Autodesk Fusion 360 part; units mm, degrees
(part 2 of 3)
sketch "스케치11" plane through (120.25, 0, 0) normal (1, 0, 0) x (0, 1, 0)
  line L0 (-4, 0) -> (79.3, 0)
  line L1 (79.3, 0) -> (79.3, 132.5)
  line L2 (79.3, 132.5) -> (-4, 132.5)
  line L3 (-4, 132.5) -> (-4, 0)
  line L4 (1, 128.5) -> (1, 4)
  line L5 (1, 4) -> (74.3, 4)
  line L6 (74.3, 4) -> (74.3, 128.5)
  line L7 (74.3, 128.5) -> (1, 128.5)
  line L8 (40.15, 61.9199) -> (42.65, 66.25)
  line L9 (42.65, 66.25) -> (40.15, 70.5801)
  line L10 (40.15, 70.5801) -> (35.15, 70.5801)
  line L11 (35.15, 70.5801) -> (32.65, 66.25)
  line L12 (32.65, 66.25) -> (35.15, 61.9199)
  line L13 (35.15, 61.9199) -> (40.15, 61.9199)
  line L14 (51.8821, 60.9199) -> (49.3821, 65.25)
  line L15 (49.3821, 65.25) -> (44.3821, 65.25)
  line L16 (44.3821, 65.25) -> (41.8821, 60.9199)
  line L17 (41.8821, 60.9199) -> (44.3821, 56.5897)
  line L18 (44.3821, 56.5897) -> (49.3821, 56.5897)
  line L19 (49.3821, 56.5897) -> (51.8821, 60.9199)
  line L20 (42.65, 66.25) -> (44.3821, 65.25) construction
  line L21 (74.3, 66.25) -> (1, 66.25) construction
  line L22 (37.65, 128.5) -> (37.65, 4) construction
  line L23 (-4, 132.5) -> (-4, 0)
  line L24 (79.3, 132.5) -> (79.3, 0)
  line L25 (79.3, 132.5) -> (-4, 132.5)
  line L26 (5.722, 2.29) -> (3.222, 6.6201)
  line L27 (7.4541, 1.29) -> (4.9541, -3.0401)
  line L28 (3.222, -2.0401) -> (5.722, 2.29)
  line L29 (3.222, 6.6201) -> (-1.778, 6.6201)
  line L30 (14.9541, -3.0401) -> (12.4541, 1.29)
  line L31 (12.4541, 1.29) -> (7.4541, 1.29)
  line L32 (7.4541, -7.3703) -> (12.4541, -7.3703)
  line L33 (12.4541, -7.3703) -> (14.9541, -3.0401)
  line L34 (-1.778, -2.0401) -> (3.222, -2.0401)
  line L35 (4.9541, -3.0401) -> (7.4541, -7.3703)
  line L36 (-1.778, 6.6201) -> (-4.278, 2.29)
  line L37 (-4.278, 2.29) -> (-1.778, -2.0401)
  line L38 (5.722, 2.29) -> (7.4541, 1.29) construction
  line L39 (24.186, 2.29) -> (21.686, 6.6201)
  line L40 (25.9181, 1.29) -> (23.4181, -3.0401)
  line L41 (21.686, -2.0401) -> (24.186, 2.29)
  line L42 (21.686, 6.6201) -> (16.686, 6.6201)
  line L43 (33.4181, -3.0401) -> (30.9181, 1.29)
  line L44 (30.9181, 1.29) -> (25.9181, 1.29)
  line L45 (25.9181, -7.3703) -> (30.9181, -7.3703)
  line L46 (30.9181, -7.3703) -> (33.4181, -3.0401)
  line L47 (16.686, -2.0401) -> (21.686, -2.0401)
  line L48 (23.4181, -3.0401) -> (25.9181, -7.3703)
  line L49 (16.686, 6.6201) -> (14.186, 2.29)
  line L50 (14.186, 2.29) -> (16.686, -2.0401)
  line L51 (24.186, 2.29) -> (25.9181, 1.29) construction
  line L52 (42.65, 2.29) -> (40.15, 6.6201)
  line L53 (44.3821, 1.29) -> (41.8821, -3.0401)
  line L54 (40.15, -2.0401) -> (42.65, 2.29)
  line L55 (40.15, 6.6201) -> (35.15, 6.6201)
  line L56 (51.8821, -3.0401) -> (49.3821, 1.29)
  line L57 (49.3821, 1.29) -> (44.3821, 1.29)
  line L58 (44.3821, -7.3703) -> (49.3821, -7.3703)
  line L59 (49.3821, -7.3703) -> (51.8821, -3.0401)
  line L60 (35.15, -2.0401) -> (40.15, -2.0401)
  line L61 (41.8821, -3.0401) -> (44.3821, -7.3703)
  line L62 (35.15, 6.6201) -> (32.65, 2.29)
  line L63 (32.65, 2.29) -> (35.15, -2.0401)
  line L64 (42.65, 2.29) -> (44.3821, 1.29) construction
  line L65 (61.114, 2.29) -> (58.614, 6.6201)
  line L66 (62.8461, 1.29) -> (60.3461, -3.0401)
  line L67 (58.614, -2.0401) -> (61.114, 2.29)
  line L68 (58.614, 6.6201) -> (53.614, 6.6201)
  line L69 (70.3461, -3.0401) -> (67.8461, 1.29)
  line L70 (67.8461, 1.29) -> (62.8461, 1.29)
  line L71 (62.8461, -7.3703) -> (67.8461, -7.3703)
  line L72 (67.8461, -7.3703) -> (70.3461, -3.0401)
  line L73 (53.614, -2.0401) -> (58.614, -2.0401)
  line L74 (60.3461, -3.0401) -> (62.8461, -7.3703)
  line L75 (53.614, 6.6201) -> (51.114, 2.29)
  line L76 (51.114, 2.29) -> (53.614, -2.0401)
  line L77 (61.114, 2.29) -> (62.8461, 1.29) construction
  line L78 (79.578, 2.29) -> (77.078, 6.6201)
  line L79 (81.3101, 1.29) -> (78.8101, -3.0401)
  line L80 (77.078, -2.0401) -> (79.578, 2.29)
  line L81 (77.078, 6.6201) -> (72.078, 6.6201)
  line L82 (88.8101, -3.0401) -> (86.3101, 1.29)
  line L83 (86.3101, 1.29) -> (81.3101, 1.29)
  line L84 (81.3101, -7.3703) -> (86.3101, -7.3703)
  line L85 (86.3101, -7.3703) -> (88.8101, -3.0401)
  line L86 (72.078, -2.0401) -> (77.078, -2.0401)
  line L87 (78.8101, -3.0401) -> (81.3101, -7.3703)
  line L88 (72.078, 6.6201) -> (69.578, 2.29)
  line L89 (69.578, 2.29) -> (72.078, -2.0401)
  line L90 (79.578, 2.29) -> (81.3101, 1.29) construction
  line L91 (5.722, 12.95) -> (3.222, 17.2801)
  line L92 (7.4541, 11.95) -> (4.9541, 7.6199)
  line L93 (3.222, 8.6199) -> (5.722, 12.95)
  line L94 (3.222, 17.2801) -> (-1.778, 17.2801)
  line L95 (14.9541, 7.6199) -> (12.4541, 11.95)
  line L96 (12.4541, 11.95) -> (7.4541, 11.95)
  line L97 (7.4541, 3.2897) -> (12.4541, 3.2897)
  line L98 (12.4541, 3.2897) -> (14.9541, 7.6199)
  line L99 (-1.778, 8.6199) -> (3.222, 8.6199)
  line L100 (4.9541, 7.6199) -> (7.4541, 3.2897)
  line L101 (-1.778, 17.2801) -> (-4.278, 12.95)
  line L102 (-4.278, 12.95) -> (-1.778, 8.6199)
  line L103 (5.722, 12.95) -> (7.4541, 11.95) construction
  line L104 (24.186, 12.95) -> (21.686, 17.2801)
  line L105 (25.9181, 11.95) -> (23.4181, 7.6199)
  line L106 (21.686, 8.6199) -> (24.186, 12.95)
  line L107 (21.686, 17.2801) -> (16.686, 17.2801)
  line L108 (33.4181, 7.6199) -> (30.9181, 11.95)
  line L109 (30.9181, 11.95) -> (25.9181, 11.95)
  line L110 (25.9181, 3.2897) -> (30.9181, 3.2897)
  line L111 (30.9181, 3.2897) -> (33.4181, 7.6199)
  line L112 (16.686, 8.6199) -> (21.686, 8.6199)
  line L113 (23.4181, 7.6199) -> (25.9181, 3.2897)
  line L114 (16.686, 17.2801) -> (14.186, 12.95)
  line L115 (14.186, 12.95) -> (16.686, 8.6199)
  line L116 (24.186, 12.95) -> (25.9181, 11.95) construction
  line L117 (42.65, 12.95) -> (40.15, 17.2801)
  line L118 (44.3821, 11.95) -> (41.8821, 7.6199)
  line L119 (40.15, 8.6199) -> (42.65, 12.95)
  line L120 (40.15, 17.2801) -> (35.15, 17.2801)
  line L121 (51.8821, 7.6199) -> (49.3821, 11.95)
  line L122 (49.3821, 11.95) -> (44.3821, 11.95)
  line L123 (44.3821, 3.2897) -> (49.3821, 3.2897)
  line L124 (49.3821, 3.2897) -> (51.8821, 7.6199)
  line L125 (35.15, 8.6199) -> (40.15, 8.6199)
  line L126 (41.8821, 7.6199) -> (44.3821, 3.2897)
  line L127 (35.15, 17.2801) -> (32.65, 12.95)
  line L128 (32.65, 12.95) -> (35.15, 8.6199)
  line L129 (42.65, 12.95) -> (44.3821, 11.95) construction
  line L130 (61.114, 12.95) -> (58.614, 17.2801)
  line L131 (62.8461, 11.95) -> (60.3461, 7.6199)
  line L132 (58.614, 8.6199) -> (61.114, 12.95)
  line L133 (58.614, 17.2801) -> (53.614, 17.2801)
  line L134 (70.3461, 7.6199) -> (67.8461, 11.95)
  line L135 (67.8461, 11.95) -> (62.8461, 11.95)
  line L136 (62.8461, 3.2897) -> (67.8461, 3.2897)
  line L137 (67.8461, 3.2897) -> (70.3461, 7.6199)
  line L138 (53.614, 8.6199) -> (58.614, 8.6199)
  line L139 (60.3461, 7.6199) -> (62.8461, 3.2897)
  line L140 (53.614, 17.2801) -> (51.114, 12.95)
  line L141 (51.114, 12.95) -> (53.614, 8.6199)
  line L142 (61.114, 12.95) -> (62.8461, 11.95) construction
  line L143 (79.578, 12.95) -> (77.078, 17.2801)
  line L144 (81.3101, 11.95) -> (78.8101, 7.6199)
  line L145 (77.078, 8.6199) -> (79.578, 12.95)
  line L146 (77.078, 17.2801) -> (72.078, 17.2801)
  line L147 (88.8101, 7.6199) -> (86.3101, 11.95)
  line L148 (86.3101, 11.95) -> (81.3101, 11.95)
  line L149 (81.3101, 3.2897) -> (86.3101, 3.2897)
  line L150 (86.3101, 3.2897) -> (88.8101, 7.6199)
  line L151 (72.078, 8.6199) -> (77.078, 8.6199)
  line L152 (78.8101, 7.6199) -> (81.3101, 3.2897)
  line L153 (72.078, 17.2801) -> (69.578, 12.95)
  line L154 (69.578, 12.95) -> (72.078, 8.6199)
  line L155 (79.578, 12.95) -> (81.3101, 11.95) construction
  line L156 (5.722, 23.61) -> (3.222, 27.9401)
  line L157 (7.4541, 22.61) -> (4.9541, 18.2799)
  line L158 (3.222, 19.2799) -> (5.722, 23.61)
  line L159 (3.222, 27.9401) -> (-1.778, 27.9401)
  line L160 (14.9541, 18.2799) -> (12.4541, 22.61)
  line L161 (12.4541, 22.61) -> (7.4541, 22.61)
  line L162 (7.4541, 13.9497) -> (12.4541, 13.9497)
  line L163 (12.4541, 13.9497) -> (14.9541, 18.2799)
  line L164 (-1.778, 19.2799) -> (3.222, 19.2799)
  line L165 (4.9541, 18.2799) -> (7.4541, 13.9497)
  line L166 (-1.778, 27.9401) -> (-4.278, 23.61)
  line L167 (-4.278, 23.61) -> (-1.778, 19.2799)
  line L168 (5.722, 23.61) -> (7.4541, 22.61) construction
  line L169 (24.186, 23.61) -> (21.686, 27.9401)
  line L170 (25.9181, 22.61) -> (23.4181, 18.2799)
  line L171 (21.686, 19.2799) -> (24.186, 23.61)
  line L172 (21.686, 27.9401) -> (16.686, 27.9401)
  line L173 (33.4181, 18.2799) -> (30.9181, 22.61)
  line L174 (30.9181, 22.61) -> (25.9181, 22.61)
  line L175 (25.9181, 13.9497) -> (30.9181, 13.9497)
  line L176 (30.9181, 13.9497) -> (33.4181, 18.2799)
  line L177 (16.686, 19.2799) -> (21.686, 19.2799)
  line L178 (23.4181, 18.2799) -> (25.9181, 13.9497)
  line L179 (16.686, 27.9401) -> (14.186, 23.61)
  line L180 (14.186, 23.61) -> (16.686, 19.2799)
  line L181 (24.186, 23.61) -> (25.9181, 22.61) construction
  line L182 (42.65, 23.61) -> (40.15, 27.9401)
  line L183 (44.3821, 22.61) -> (41.8821, 18.2799)
  line L184 (40.15, 19.2799) -> (42.65, 23.61)
  line L185 (40.15, 27.9401) -> (35.15, 27.9401)
  line L186 (51.8821, 18.2799) -> (49.3821, 22.61)
  line L187 (49.3821, 22.61) -> (44.3821, 22.61)
  line L188 (44.3821, 13.9497) -> (49.3821, 13.9497)
  line L189 (49.3821, 13.9497) -> (51.8821, 18.2799)
  line L190 (35.15, 19.2799) -> (40.15, 19.2799)
  line L191 (41.8821, 18.2799) -> (44.3821, 13.9497)
  line L192 (35.15, 27.9401) -> (32.65, 23.61)
  line L193 (32.65, 23.61) -> (35.15, 19.2799)
  line L194 (42.65, 23.61) -> (44.3821, 22.61) construction
  line L195 (61.114, 23.61) -> (58.614, 27.9401)
  line L196 (62.8461, 22.61) -> (60.3461, 18.2799)
  line L197 (58.614, 19.2799) -> (61.114, 23.61)
  line L198 (58.614, 27.9401) -> (53.614, 27.9401)
  line L199 (70.3461, 18.2799) -> (67.8461, 22.61)
  line L200 (67.8461, 22.61) -> (62.8461, 22.61)
  line L201 (62.8461, 13.9497) -> (67.8461, 13.9497)
  line L202 (67.8461, 13.9497) -> (70.3461, 18.2799)
  line L203 (53.614, 19.2799) -> (58.614, 19.2799)
  line L204 (60.3461, 18.2799) -> (62.8461, 13.9497)
  line L205 (53.614, 27.9401) -> (51.114, 23.61)
  line L206 (51.114, 23.61) -> (53.614, 19.2799)
  line L207 (61.114, 23.61) -> (62.8461, 22.61) construction
  line L208 (79.578, 23.61) -> (77.078, 27.9401)
  line L209 (81.3101, 22.61) -> (78.8101, 18.2799)
  line L210 (77.078, 19.2799) -> (79.578, 23.61)
  line L211 (77.078, 27.9401) -> (72.078, 27.9401)
  line L212 (88.8101, 18.2799) -> (86.3101, 22.61)
  line L213 (86.3101, 22.61) -> (81.3101, 22.61)
  line L214 (81.3101, 13.9497) -> (86.3101, 13.9497)
  line L215 (86.3101, 13.9497) -> (88.8101, 18.2799)
  line L216 (72.078, 19.2799) -> (77.078, 19.2799)
  line L217 (78.8101, 18.2799) -> (81.3101, 13.9497)
  line L218 (72.078, 27.9401) -> (69.578, 23.61)
  line L219 (69.578, 23.61) -> (72.078, 19.2799)
  line L220 (79.578, 23.61) -> (81.3101, 22.61) construction
  line L221 (5.722, 34.27) -> (3.222, 38.6001)
  line L222 (7.4541, 33.27) -> (4.9541, 28.9399)
  line L223 (3.222, 29.9399) -> (5.722, 34.27)
  line L224 (3.222, 38.6001) -> (-1.778, 38.6001)
  line L225 (14.9541, 28.9399) -> (12.4541, 33.27)
  line L226 (12.4541, 33.27) -> (7.4541, 33.27)
  line L227 (7.4541, 24.6097) -> (12.4541, 24.6097)
  line L228 (12.4541, 24.6097) -> (14.9541, 28.9399)
  line L229 (-1.778, 29.9399) -> (3.222, 29.9399)
  line L230 (4.9541, 28.9399) -> (7.4541, 24.6097)
  line L231 (-1.778, 38.6001) -> (-4.278, 34.27)
  line L232 (-4.278, 34.27) -> (-1.778, 29.9399)
  line L233 (5.722, 34.27) -> (7.4541, 33.27) construction
  line L234 (24.186, 34.27) -> (21.686, 38.6001)
  line L235 (25.9181, 33.27) -> (23.4181, 28.9399)
  line L236 (21.686, 29.9399) -> (24.186, 34.27)
  line L237 (21.686, 38.6001) -> (16.686, 38.6001)
  line L238 (33.4181, 28.9399) -> (30.9181, 33.27)
  line L239 (30.9181, 33.27) -> (25.9181, 33.27)
  line L240 (25.9181, 24.6097) -> (30.9181, 24.6097)
  line L241 (30.9181, 24.6097) -> (33.4181, 28.9399)
  line L242 (16.686, 29.9399) -> (21.686, 29.9399)
  line L243 (23.4181, 28.9399) -> (25.9181, 24.6097)
  line L244 (16.686, 38.6001) -> (14.186, 34.27)
  line L245 (14.186, 34.27) -> (16.686, 29.9399)
  line L246 (24.186, 34.27) -> (25.9181, 33.27) construction
  line L247 (42.65, 34.27) -> (40.15, 38.6001)
  line L248 (44.3821, 33.27) -> (41.8821, 28.9399)
  line L249 (40.15, 29.9399) -> (42.65, 34.27)
  line L250 (40.15, 38.6001) -> (35.15, 38.6001)
  line L251 (51.8821, 28.9399) -> (49.3821, 33.27)
  line L252 (49.3821, 33.27) -> (44.3821, 33.27)
  line L253 (44.3821, 24.6097) -> (49.3821, 24.6097)
  line L254 (49.3821, 24.6097) -> (51.8821, 28.9399)
  line L255 (35.15, 29.9399) -> (40.15, 29.9399)
  line L256 (41.8821, 28.9399) -> (44.3821, 24.6097)
  line L257 (35.15, 38.6001) -> (32.65, 34.27)
  line L258 (32.65, 34.27) -> (35.15, 29.9399)
  line L259 (42.65, 34.27) -> (44.3821, 33.27) construction
  line L260 (61.114, 34.27) -> (58.614, 38.6001)
  line L261 (62.8461, 33.27) -> (60.3461, 28.9399)
  line L262 (58.614, 29.9399) -> (61.114, 34.27)
  line L263 (58.614, 38.6001) -> (53.614, 38.6001)
  line L264 (70.3461, 28.9399) -> (67.8461, 33.27)
  line L265 (67.8461, 33.27) -> (62.8461, 33.27)
  line L266 (62.8461, 24.6097) -> (67.8461, 24.6097)
  line L267 (67.8461, 24.6097) -> (70.3461, 28.9399)
  line L268 (53.614, 29.9399) -> (58.614, 29.9399)
  line L269 (60.3461, 28.9399) -> (62.8461, 24.6097)
  line L270 (53.614, 38.6001) -> (51.114, 34.27)
  line L271 (51.114, 34.27) -> (53.614, 29.9399)
  line L272 (61.114, 34.27) -> (62.8461, 33.27) construction
  line L273 (79.578, 34.27) -> (77.078, 38.6001)
  line L274 (81.3101, 33.27) -> (78.8101, 28.9399)
  line L275 (77.078, 29.9399) -> (79.578, 34.27)
  line L276 (77.078, 38.6001) -> (72.078, 38.6001)
  line L277 (88.8101, 28.9399) -> (86.3101, 33.27)
  line L278 (86.3101, 33.27) -> (81.3101, 33.27)
  line L279 (81.3101, 24.6097) -> (86.3101, 24.6097)
  line L280 (86.3101, 24.6097) -> (88.8101, 28.9399)
  line L281 (72.078, 29.9399) -> (77.078, 29.9399)
  line L282 (78.8101, 28.9399) -> (81.3101, 24.6097)
  line L283 (72.078, 38.6001) -> (69.578, 34.27)
  line L284 (69.578, 34.27) -> (72.078, 29.9399)
  line L285 (79.578, 34.27) -> (81.3101, 33.27) construction
  line L286 (5.722, 44.93) -> (3.222, 49.2601)
  line L287 (7.4541, 43.93) -> (4.9541, 39.5999)
  line L288 (3.222, 40.5999) -> (5.722, 44.93)
  line L289 (3.222, 49.2601) -> (-1.778, 49.2601)
  line L290 (14.9541, 39.5999) -> (12.4541, 43.93)
  line L291 (12.4541, 43.93) -> (7.4541, 43.93)
  line L292 (7.4541, 35.2697) -> (12.4541, 35.2697)
  line L293 (12.4541, 35.2697) -> (14.9541, 39.5999)
  line L294 (-1.778, 40.5999) -> (3.222, 40.5999)
  line L295 (4.9541, 39.5999) -> (7.4541, 35.2697)
  line L296 (-1.778, 49.2601) -> (-4.278, 44.93)
  line L297 (-4.278, 44.93) -> (-1.778, 40.5999)
  line L298 (5.722, 44.93) -> (7.4541, 43.93) construction
  line L299 (24.186, 44.93) -> (21.686, 49.2601)
  line L300 (25.9181, 43.93) -> (23.4181, 39.5999)
  line L301 (21.686, 40.5999) -> (24.186, 44.93)
  line L302 (21.686, 49.2601) -> (16.686, 49.2601)
  line L303 (33.4181, 39.5999) -> (30.9181, 43.93)
  line L304 (30.9181, 43.93) -> (25.9181, 43.93)
  line L305 (25.9181, 35.2697) -> (30.9181, 35.2697)
  line L306 (30.9181, 35.2697) -> (33.4181, 39.5999)
  line L307 (16.686, 40.5999) -> (21.686, 40.5999)
  line L308 (23.4181, 39.5999) -> (25.9181, 35.2697)
  line L309 (16.686, 49.2601) -> (14.186, 44.93)
  line L310 (14.186, 44.93) -> (16.686, 40.5999)
  line L311 (24.186, 44.93) -> (25.9181, 43.93) construction
  line L312 (42.65, 44.93) -> (40.15, 49.2601)
  line L313 (44.3821, 43.93) -> (41.8821, 39.5999)
  line L314 (40.15, 40.5999) -> (42.65, 44.93)
  line L315 (40.15, 49.2601) -> (35.15, 49.2601)
  line L316 (51.8821, 39.5999) -> (49.3821, 43.93)
  line L317 (49.3821, 43.93) -> (44.3821, 43.93)
  line L318 (44.3821, 35.2697) -> (49.3821, 35.2697)
  line L319 (49.3821, 35.2697) -> (51.8821, 39.5999)
  line L320 (35.15, 40.5999) -> (40.15, 40.5999)
  line L321 (41.8821, 39.5999) -> (44.3821, 35.2697)
  line L322 (35.15, 49.2601) -> (32.65, 44.93)
  line L323 (32.65, 44.93) -> (35.15, 40.5999)
  line L324 (42.65, 44.93) -> (44.3821, 43.93) construction
  line L325 (61.114, 44.93) -> (58.614, 49.2601)
  line L326 (62.8461, 43.93) -> (60.3461, 39.5999)
  line L327 (58.614, 40.5999) -> (61.114, 44.93)
  line L328 (58.614, 49.2601) -> (53.614, 49.2601)
  line L329 (70.3461, 39.5999) -> (67.8461, 43.93)
  line L330 (67.8461, 43.93) -> (62.8461, 43.93)
  line L331 (62.8461, 35.2697) -> (67.8461, 35.2697)
  line L332 (67.8461, 35.2697) -> (70.3461, 39.5999)
  line L333 (53.614, 40.5999) -> (58.614, 40.5999)
  line L334 (60.3461, 39.5999) -> (62.8461, 35.2697)
  line L335 (53.614, 49.2601) -> (51.114, 44.93)
  line L336 (51.114, 44.93) -> (53.614, 40.5999)
  line L337 (61.114, 44.93) -> (62.8461, 43.93) construction
  line L338 (79.578, 44.93) -> (77.078, 49.2601)
  line L339 (81.3101, 43.93) -> (78.8101, 39.5999)
  line L340 (77.078, 40.5999) -> (79.578, 44.93)
  line L341 (77.078, 49.2601) -> (72.078, 49.2601)
  line L342 (88.8101, 39.5999) -> (86.3101, 43.93)
  line L343 (86.3101, 43.93) -> (81.3101, 43.93)
  line L344 (81.3101, 35.2697) -> (86.3101, 35.2697)
  line L345 (86.3101, 35.2697) -> (88.8101, 39.5999)
  line L346 (72.078, 40.5999) -> (77.078, 40.5999)
  line L347 (78.8101, 39.5999) -> (81.3101, 35.2697)
  line L348 (72.078, 49.2601) -> (69.578, 44.93)
  line L349 (69.578, 44.93) -> (72.078, 40.5999)
  line L350 (79.578, 44.93) -> (81.3101, 43.93) construction
  line L351 (5.722, 55.59) -> (3.222, 59.9201)
  line L352 (7.4541, 54.59) -> (4.9541, 50.2599)
  line L353 (3.222, 51.2599) -> (5.722, 55.59)
  line L354 (3.222, 59.9201) -> (-1.778, 59.9201)
  line L355 (14.9541, 50.2599) -> (12.4541, 54.59)
  line L356 (12.4541, 54.59) -> (7.4541, 54.59)
  line L357 (7.4541, 45.9297) -> (12.4541, 45.9297)
  line L358 (12.4541, 45.9297) -> (14.9541, 50.2599)
  line L359 (-1.778, 51.2599) -> (3.222, 51.2599)
  line L360 (4.9541, 50.2599) -> (7.4541, 45.9297)
  line L361 (-1.778, 59.9201) -> (-4.278, 55.59)
  line L362 (-4.278, 55.59) -> (-1.778, 51.2599)
  line L363 (5.722, 55.59) -> (7.4541, 54.59) construction
  line L364 (24.186, 55.59) -> (21.686, 59.9201)
  line L365 (25.9181, 54.59) -> (23.4181, 50.2599)
  line L366 (21.686, 51.2599) -> (24.186, 55.59)
  line L367 (21.686, 59.9201) -> (16.686, 59.9201)
  line L368 (33.4181, 50.2599) -> (30.9181, 54.59)
  line L369 (30.9181, 54.59) -> (25.9181, 54.59)
  line L370 (25.9181, 45.9297) -> (30.9181, 45.9297)
  line L371 (30.9181, 45.9297) -> (33.4181, 50.2599)
  line L372 (16.686, 51.2599) -> (21.686, 51.2599)
  line L373 (23.4181, 50.2599) -> (25.9181, 45.9297)
  line L374 (16.686, 59.9201) -> (14.186, 55.59)
  line L375 (14.186, 55.59) -> (16.686, 51.2599)
  line L376 (24.186, 55.59) -> (25.9181, 54.59) construction
  line L377 (42.65, 55.59) -> (40.15, 59.9201)
  line L378 (44.3821, 54.59) -> (41.8821, 50.2599)
  line L379 (40.15, 51.2599) -> (42.65, 55.59)
  line L380 (40.15, 59.9201) -> (35.15, 59.9201)
  line L381 (51.8821, 50.2599) -> (49.3821, 54.59)
  line L382 (49.3821, 54.59) -> (44.3821, 54.59)
  line L383 (44.3821, 45.9297) -> (49.3821, 45.9297)
  line L384 (49.3821, 45.9297) -> (51.8821, 50.2599)
  line L385 (35.15, 51.2599) -> (40.15, 51.2599)
  line L386 (41.8821, 50.2599) -> (44.3821, 45.9297)
  line L387 (35.15, 59.9201) -> (32.65, 55.59)
  line L388 (32.65, 55.59) -> (35.15, 51.2599)
  line L389 (42.65, 55.59) -> (44.3821, 54.59) construction
  line L390 (61.114, 55.59) -> (58.614, 59.9201)
  line L391 (62.8461, 54.59) -> (60.3461, 50.2599)
  line L392 (58.614, 51.2599) -> (61.114, 55.59)
  line L393 (58.614, 59.9201) -> (53.614, 59.9201)
  line L394 (70.3461, 50.2599) -> (67.8461, 54.59)
  line L395 (67.8461, 54.59) -> (62.8461, 54.59)
  line L396 (62.8461, 45.9297) -> (67.8461, 45.9297)
  line L397 (67.8461, 45.9297) -> (70.3461, 50.2599)
  line L398 (53.614, 51.2599) -> (58.614, 51.2599)
  line L399 (60.3461, 50.2599) -> (62.8461, 45.9297)
  line L400 (53.614, 59.9201) -> (51.114, 55.59)
  line L401 (51.114, 55.59) -> (53.614, 51.2599)
  line L402 (61.114, 55.59) -> (62.8461, 54.59) construction
  line L403 (79.578, 55.59) -> (77.078, 59.9201)
  line L404 (81.3101, 54.59) -> (78.8101, 50.2599)
  line L405 (77.078, 51.2599) -> (79.578, 55.59)
  line L406 (77.078, 59.9201) -> (72.078, 59.9201)
  line L407 (88.8101, 50.2599) -> (86.3101, 54.59)
  line L408 (86.3101, 54.59) -> (81.3101, 54.59)
  line L409 (81.3101, 45.9297) -> (86.3101, 45.9297)
  line L410 (86.3101, 45.9297) -> (88.8101, 50.2599)
  line L411 (72.078, 51.2599) -> (77.078, 51.2599)
  line L412 (78.8101, 50.2599) -> (81.3101, 45.9297)
  line L413 (72.078, 59.9201) -> (69.578, 55.59)
  line L414 (69.578, 55.59) -> (72.078, 51.2599)
  line L415 (79.578, 55.59) -> (81.3101, 54.59) construction
  line L416 (5.722, 66.25) -> (3.222, 70.5801)
  line L417 (7.4541, 65.25) -> (4.9541, 60.9199)
  line L418 (3.222, 61.9199) -> (5.722, 66.25)
  line L419 (3.222, 70.5801) -> (-1.778, 70.5801)
  line L420 (14.9541, 60.9199) -> (12.4541, 65.25)
  line L421 (12.4541, 65.25) -> (7.4541, 65.25)
  line L422 (7.4541, 56.5897) -> (12.4541, 56.5897)
  line L423 (12.4541, 56.5897) -> (14.9541, 60.9199)
  line L424 (-1.778, 61.9199) -> (3.222, 61.9199)
  line L425 (4.9541, 60.9199) -> (7.4541, 56.5897)
  line L426 (-1.778, 70.5801) -> (-4.278, 66.25)
  line L427 (-4.278, 66.25) -> (-1.778, 61.9199)
  line L428 (5.722, 66.25) -> (7.4541, 65.25) construction
  line L429 (24.186, 66.25) -> (21.686, 70.5801)
  line L430 (25.9181, 65.25) -> (23.4181, 60.9199)
  line L431 (21.686, 61.9199) -> (24.186, 66.25)
  line L432 (21.686, 70.5801) -> (16.686, 70.5801)
  line L433 (33.4181, 60.9199) -> (30.9181, 65.25)
  line L434 (30.9181, 65.25) -> (25.9181, 65.25)
  line L435 (25.9181, 56.5897) -> (30.9181, 56.5897)
  line L436 (30.9181, 56.5897) -> (33.4181, 60.9199)
  line L437 (16.686, 61.9199) -> (21.686, 61.9199)
  line L438 (23.4181, 60.9199) -> (25.9181, 56.5897)
  line L439 (16.686, 70.5801) -> (14.186, 66.25)
  line L440 (14.186, 66.25) -> (16.686, 61.9199)
  line L441 (24.186, 66.25) -> (25.9181, 65.25) construction
  line L442 (61.114, 66.25) -> (58.614, 70.5801)
  line L443 (62.8461, 65.25) -> (60.3461, 60.9199)
  line L444 (58.614, 61.9199) -> (61.114, 66.25)
  line L445 (58.614, 70.5801) -> (53.614, 70.5801)
  line L446 (70.3461, 60.9199) -> (67.8461, 65.25)
  line L447 (67.8461, 65.25) -> (62.8461, 65.25)
  line L448 (62.8461, 56.5897) -> (67.8461, 56.5897)
  line L449 (67.8461, 56.5897) -> (70.3461, 60.9199)
  line L450 (53.614, 61.9199) -> (58.614, 61.9199)
  line L451 (60.3461, 60.9199) -> (62.8461, 56.5897)
  line L452 (53.614, 70.5801) -> (51.114, 66.25)
  line L453 (51.114, 66.25) -> (53.614, 61.9199)
  line L454 (61.114, 66.25) -> (62.8461, 65.25) construction
  line L455 (79.578, 66.25) -> (77.078, 70.5801)
  line L456 (81.3101, 65.25) -> (78.8101, 60.9199)
  line L457 (77.078, 61.9199) -> (79.578, 66.25)
  line L458 (77.078, 70.5801) -> (72.078, 70.5801)
  line L459 (88.8101, 60.9199) -> (86.3101, 65.25)
  line L460 (86.3101, 65.25) -> (81.3101, 65.25)
  line L461 (81.3101, 56.5897) -> (86.3101, 56.5897)
  line L462 (86.3101, 56.5897) -> (88.8101, 60.9199)
  line L463 (72.078, 61.9199) -> (77.078, 61.9199)
  line L464 (78.8101, 60.9199) -> (81.3101, 56.5897)
  line L465 (72.078, 70.5801) -> (69.578, 66.25)
  line L466 (69.578, 66.25) -> (72.078, 61.9199)
  line L467 (79.578, 66.25) -> (81.3101, 65.25) construction
  line L468 (5.722, 76.91) -> (3.222, 81.2401)
  line L469 (7.4541, 75.91) -> (4.9541, 71.5799)
  line L470 (3.222, 72.5799) -> (5.722, 76.91)
  line L471 (3.222, 81.2401) -> (-1.778, 81.2401)
  line L472 (14.9541, 71.5799) -> (12.4541, 75.91)
  line L473 (12.4541, 75.91) -> (7.4541, 75.91)
  line L474 (7.4541, 67.2497) -> (12.4541, 67.2497)
  line L475 (12.4541, 67.2497) -> (14.9541, 71.5799)
  line L476 (-1.778, 72.5799) -> (3.222, 72.5799)
  line L477 (4.9541, 71.5799) -> (7.4541, 67.2497)
  line L478 (-1.778, 81.2401) -> (-4.278, 76.91)
  line L479 (-4.278, 76.91) -> (-1.778, 72.5799)
  line L480 (5.722, 76.91) -> (7.4541, 75.91) construction
  line L481 (24.186, 76.91) -> (21.686, 81.2401)
  line L482 (25.9181, 75.91) -> (23.4181, 71.5799)
  line L483 (21.686, 72.5799) -> (24.186, 76.91)
  line L484 (21.686, 81.2401) -> (16.686, 81.2401)
  line L485 (33.4181, 71.5799) -> (30.9181, 75.91)
  line L486 (30.9181, 75.91) -> (25.9181, 75.91)
  line L487 (25.9181, 67.2497) -> (30.9181, 67.2497)
  line L488 (30.9181, 67.2497) -> (33.4181, 71.5799)
  line L489 (16.686, 72.5799) -> (21.686, 72.5799)
  line L490 (23.4181, 71.5799) -> (25.9181, 67.2497)
  line L491 (16.686, 81.2401) -> (14.186, 76.91)
  line L492 (14.186, 76.91) -> (16.686, 72.5799)
  line L493 (24.186, 76.91) -> (25.9181, 75.91) construction
  line L494 (42.65, 76.91) -> (40.15, 81.2401)
  line L495 (44.3821, 75.91) -> (41.8821, 71.5799)
  line L496 (40.15, 72.5799) -> (42.65, 76.91)
  line L497 (40.15, 81.2401) -> (35.15, 81.2401)
  line L498 (51.8821, 71.5799) -> (49.3821, 75.91)
  line L499 (49.3821, 75.91) -> (44.3821, 75.91)
  line L500 (44.3821, 67.2497) -> (49.3821, 67.2497)
  line L501 (49.3821, 67.2497) -> (51.8821, 71.5799)
  line L502 (35.15, 72.5799) -> (40.15, 72.5799)
  line L503 (41.8821, 71.5799) -> (44.3821, 67.2497)
  line L504 (35.15, 81.2401) -> (32.65, 76.91)
  line L505 (32.65, 76.91) -> (35.15, 72.5799)
  line L506 (42.65, 76.91) -> (44.3821, 75.91) construction
  line L507 (61.114, 76.91) -> (58.614, 81.2401)
  line L508 (62.8461, 75.91) -> (60.3461, 71.5799)
  line L509 (58.614, 72.5799) -> (61.114, 76.91)
  line L510 (58.614, 81.2401) -> (53.614, 81.2401)
  line L511 (70.3461, 71.5799) -> (67.8461, 75.91)
  line L512 (67.8461, 75.91) -> (62.8461, 75.91)
  line L513 (62.8461, 67.2497) -> (67.8461, 67.2497)
  line L514 (67.8461, 67.2497) -> (70.3461, 71.5799)
  line L515 (53.614, 72.5799) -> (58.614, 72.5799)
  line L516 (60.3461, 71.5799) -> (62.8461, 67.2497)
  line L517 (53.614, 81.2401) -> (51.114, 76.91)
  line L518 (51.114, 76.91) -> (53.614, 72.5799)
  line L519 (61.114, 76.91) -> (62.8461, 75.91) construction
  line L520 (79.578, 76.91) -> (77.078, 81.2401)
  line L521 (81.3101, 75.91) -> (78.8101, 71.5799)
  line L522 (77.078, 72.5799) -> (79.578, 76.91)
  line L523 (77.078, 81.2401) -> (72.078, 81.2401)
  line L524 (88.8101, 71.5799) -> (86.3101, 75.91)
  line L525 (86.3101, 75.91) -> (81.3101, 75.91)
  line L526 (81.3101, 67.2497) -> (86.3101, 67.2497)
  line L527 (86.3101, 67.2497) -> (88.8101, 71.5799)
  line L528 (72.078, 72.5799) -> (77.078, 72.5799)
  line L529 (78.8101, 71.5799) -> (81.3101, 67.2497)
  line L530 (72.078, 81.2401) -> (69.578, 76.91)
  line L531 (69.578, 76.91) -> (72.078, 72.5799)
  line L532 (79.578, 76.91) -> (81.3101, 75.91) construction
  line L533 (5.722, 87.57) -> (3.222, 91.9001)
  line L534 (7.4541, 86.57) -> (4.9541, 82.2399)
  line L535 (3.222, 83.2399) -> (5.722, 87.57)
  line L536 (3.222, 91.9001) -> (-1.778, 91.9001)
  line L537 (14.9541, 82.2399) -> (12.4541, 86.57)
  line L538 (12.4541, 86.57) -> (7.4541, 86.57)
  line L539 (7.4541, 77.9097) -> (12.4541, 77.9097)
  line L540 (12.4541, 77.9097) -> (14.9541, 82.2399)
  line L541 (-1.778, 83.2399) -> (3.222, 83.2399)
  line L542 (4.9541, 82.2399) -> (7.4541, 77.9097)
  line L543 (-1.778, 91.9001) -> (-4.278, 87.57)
  line L544 (-4.278, 87.57) -> (-1.778, 83.2399)
  line L545 (5.722, 87.57) -> (7.4541, 86.57) construction
  line L546 (24.186, 87.57) -> (21.686, 91.9001)
  line L547 (25.9181, 86.57) -> (23.4181, 82.2399)
  line L548 (21.686, 83.2399) -> (24.186, 87.57)
  line L549 (21.686, 91.9001) -> (16.686, 91.9001)
  line L550 (33.4181, 82.2399) -> (30.9181, 86.57)
  line L551 (30.9181, 86.57) -> (25.9181, 86.57)
  line L552 (25.9181, 77.9097) -> (30.9181, 77.9097)
  line L553 (30.9181, 77.9097) -> (33.4181, 82.2399)
  line L554 (16.686, 83.2399) -> (21.686, 83.2399)
  line L555 (23.4181, 82.2399) -> (25.9181, 77.9097)
  line L556 (16.686, 91.9001) -> (14.186, 87.57)
  line L557 (14.186, 87.57) -> (16.686, 83.2399)
  line L558 (24.186, 87.57) -> (25.9181, 86.57) construction
  line L559 (42.65, 87.57) -> (40.15, 91.9001)
  line L560 (44.3821, 86.57) -> (41.8821, 82.2399)
  line L561 (40.15, 83.2399) -> (42.65, 87.57)
  line L562 (40.15, 91.9001) -> (35.15, 91.9001)
  line L563 (51.8821, 82.2399) -> (49.3821, 86.57)
  line L564 (49.3821, 86.57) -> (44.3821, 86.57)
  line L565 (44.3821, 77.9097) -> (49.3821, 77.9097)
  line L566 (49.3821, 77.9097) -> (51.8821, 82.2399)
  line L567 (35.15, 83.2399) -> (40.15, 83.2399)
  line L568 (41.8821, 82.2399) -> (44.3821, 77.9097)
  line L569 (35.15, 91.9001) -> (32.65, 87.57)
  line L570 (32.65, 87.57) -> (35.15, 83.2399)
  line L571 (42.65, 87.57) -> (44.3821, 86.57) construction
  line L572 (61.114, 87.57) -> (58.614, 91.9001)
  line L573 (62.8461, 86.57) -> (60.3461, 82.2399)
  line L574 (58.614, 83.2399) -> (61.114, 87.57)
  line L575 (58.614, 91.9001) -> (53.614, 91.9001)
  line L576 (70.3461, 82.2399) -> (67.8461, 86.57)
  line L577 (67.8461, 86.57) -> (62.8461, 86.57)
  line L578 (62.8461, 77.9097) -> (67.8461, 77.9097)
  line L579 (67.8461, 77.9097) -> (70.3461, 82.2399)
  line L580 (53.614, 83.2399) -> (58.614, 83.2399)
  line L581 (60.3461, 82.2399) -> (62.8461, 77.9097)
  line L582 (53.614, 91.9001) -> (51.114, 87.57)
  line L583 (51.114, 87.57) -> (53.614, 83.2399)
  line L584 (61.114, 87.57) -> (62.8461, 86.57) construction
  line L585 (79.578, 87.57) -> (77.078, 91.9001)
  line L586 (81.3101, 86.57) -> (78.8101, 82.2399)
  line L587 (77.078, 83.2399) -> (79.578, 87.57)
  line L588 (77.078, 91.9001) -> (72.078, 91.9001)
  line L589 (88.8101, 82.2399) -> (86.3101, 86.57)
  line L590 (86.3101, 86.57) -> (81.3101, 86.57)
  line L591 (81.3101, 77.9097) -> (86.3101, 77.9097)
  line L592 (86.3101, 77.9097) -> (88.8101, 82.2399)
  line L593 (72.078, 83.2399) -> (77.078, 83.2399)
  line L594 (78.8101, 82.2399) -> (81.3101, 77.9097)
  line L595 (72.078, 91.9001) -> (69.578, 87.57)
  line L596 (69.578, 87.57) -> (72.078, 83.2399)
  line L597 (79.578, 87.57) -> (81.3101, 86.57) construction
  line L598 (5.722, 98.23) -> (3.222, 102.5601)
  line L599 (7.4541, 97.23) -> (4.9541, 92.8999)
  line L600 (3.222, 93.8999) -> (5.722, 98.23)
  line L601 (3.222, 102.5601) -> (-1.778, 102.5601)
  line L602 (14.9541, 92.8999) -> (12.4541, 97.23)
  line L603 (12.4541, 97.23) -> (7.4541, 97.23)
  line L604 (7.4541, 88.5697) -> (12.4541, 88.5697)
  line L605 (12.4541, 88.5697) -> (14.9541, 92.8999)
  line L606 (-1.778, 93.8999) -> (3.222, 93.8999)
  line L607 (4.9541, 92.8999) -> (7.4541, 88.5697)
  line L608 (-1.778, 102.5601) -> (-4.278, 98.23)
  line L609 (-4.278, 98.23) -> (-1.778, 93.8999)
  line L610 (5.722, 98.23) -> (7.4541, 97.23) construction
  line L611 (24.186, 98.23) -> (21.686, 102.5601)
  line L612 (25.9181, 97.23) -> (23.4181, 92.8999)
  line L613 (21.686, 93.8999) -> (24.186, 98.23)
  line L614 (21.686, 102.5601) -> (16.686, 102.5601)
  line L615 (33.4181, 92.8999) -> (30.9181, 97.23)
  line L616 (30.9181, 97.23) -> (25.9181, 97.23)
  line L617 (25.9181, 88.5697) -> (30.9181, 88.5697)
  line L618 (30.9181, 88.5697) -> (33.4181, 92.8999)
  line L619 (16.686, 93.8999) -> (21.686, 93.8999)
  line L620 (23.4181, 92.8999) -> (25.9181, 88.5697)
  line L621 (16.686, 102.5601) -> (14.186, 98.23)
  line L622 (14.186, 98.23) -> (16.686, 93.8999)
  line L623 (24.186, 98.23) -> (25.9181, 97.23) construction
  line L624 (42.65, 98.23) -> (40.15, 102.5601)
  line L625 (44.3821, 97.23) -> (41.8821, 92.8999)
  line L626 (40.15, 93.8999) -> (42.65, 98.23)
  line L627 (40.15, 102.5601) -> (35.15, 102.5601)
  line L628 (51.8821, 92.8999) -> (49.3821, 97.23)
  line L629 (49.3821, 97.23) -> (44.3821, 97.23)
  line L630 (44.3821, 88.5697) -> (49.3821, 88.5697)
  line L631 (49.3821, 88.5697) -> (51.8821, 92.8999)
  line L632 (35.15, 93.8999) -> (40.15, 93.8999)
  line L633 (41.8821, 92.8999) -> (44.3821, 88.5697)
  line L634 (35.15, 102.5601) -> (32.65, 98.23)
  line L635 (32.65, 98.23) -> (35.15, 93.8999)
  line L636 (42.65, 98.23) -> (44.3821, 97.23) construction
  line L637 (61.114, 98.23) -> (58.614, 102.5601)
  line L638 (62.8461, 97.23) -> (60.3461, 92.8999)
  line L639 (58.614, 93.8999) -> (61.114, 98.23)
  line L640 (58.614, 102.5601) -> (53.614, 102.5601)
  line L641 (70.3461, 92.8999) -> (67.8461, 97.23)
  line L642 (67.8461, 97.23) -> (62.8461, 97.23)
  line L643 (62.8461, 88.5697) -> (67.8461, 88.5697)
  line L644 (67.8461, 88.5697) -> (70.3461, 92.8999)
  line L645 (53.614, 93.8999) -> (58.614, 93.8999)
  line L646 (60.3461, 92.8999) -> (62.8461, 88.5697)
  line L647 (53.614, 102.5601) -> (51.114, 98.23)
  line L648 (51.114, 98.23) -> (53.614, 93.8999)
  line L649 (61.114, 98.23) -> (62.8461, 97.23) construction
  line L650 (79.578, 98.23) -> (77.078, 102.5601)
  line L651 (81.3101, 97.23) -> (78.8101, 92.8999)
  line L652 (77.078, 93.8999) -> (79.578, 98.23)
  line L653 (77.078, 102.5601) -> (72.078, 102.5601)
  line L654 (88.8101, 92.8999) -> (86.3101, 97.23)
  line L655 (86.3101, 97.23) -> (81.3101, 97.23)
  line L656 (81.3101, 88.5697) -> (86.3101, 88.5697)
  line L657 (86.3101, 88.5697) -> (88.8101, 92.8999)
  line L658 (72.078, 93.8999) -> (77.078, 93.8999)
  line L659 (78.8101, 92.8999) -> (81.3101, 88.5697)
  line L660 (72.078, 102.5601) -> (69.578, 98.23)
  line L661 (69.578, 98.23) -> (72.078, 93.8999)
  line L662 (79.578, 98.23) -> (81.3101, 97.23) construction
  line L663 (5.722, 108.89) -> (3.222, 113.2201)
  line L664 (7.4541, 107.89) -> (4.9541, 103.5599)
  line L665 (3.222, 104.5599) -> (5.722, 108.89)
  line L666 (3.222, 113.2201) -> (-1.778, 113.2201)
  line L667 (14.9541, 103.5599) -> (12.4541, 107.89)
  line L668 (12.4541, 107.89) -> (7.4541, 107.89)
  line L669 (7.4541, 99.2297) -> (12.4541, 99.2297)
  line L670 (12.4541, 99.2297) -> (14.9541, 103.5599)
  line L671 (-1.778, 104.5599) -> (3.222, 104.5599)
  line L672 (4.9541, 103.5599) -> (7.4541, 99.2297)
  line L673 (-1.778, 113.2201) -> (-4.278, 108.89)
  line L674 (-4.278, 108.89) -> (-1.778, 104.5599)
  line L675 (5.722, 108.89) -> (7.4541, 107.89) construction
  line L676 (24.186, 108.89) -> (21.686, 113.2201)
  line L677 (25.9181, 107.89) -> (23.4181, 103.5599)
  line L678 (21.686, 104.5599) -> (24.186, 108.89)
  line L679 (21.686, 113.2201) -> (16.686, 113.2201)
  line L680 (33.4181, 103.5599) -> (30.9181, 107.89)
  line L681 (30.9181, 107.89) -> (25.9181, 107.89)
  line L682 (25.9181, 99.2297) -> (30.9181, 99.2297)
  line L683 (30.9181, 99.2297) -> (33.4181, 103.5599)
  line L684 (16.686, 104.5599) -> (21.686, 104.5599)
  line L685 (23.4181, 103.5599) -> (25.9181, 99.2297)
  line L686 (16.686, 113.2201) -> (14.186, 108.89)
  line L687 (14.186, 108.89) -> (16.686, 104.5599)
  line L688 (24.186, 108.89) -> (25.9181, 107.89) construction
  line L689 (42.65, 108.89) -> (40.15, 113.2201)
  line L690 (44.3821, 107.89) -> (41.8821, 103.5599)
  line L691 (40.15, 104.5599) -> (42.65, 108.89)
  line L692 (40.15, 113.2201) -> (35.15, 113.2201)
  line L693 (51.8821, 103.5599) -> (49.3821, 107.89)
  line L694 (49.3821, 107.89) -> (44.3821, 107.89)
  line L695 (44.3821, 99.2297) -> (49.3821, 99.2297)
  line L696 (49.3821, 99.2297) -> (51.8821, 103.5599)
  line L697 (35.15, 104.5599) -> (40.15, 104.5599)
  line L698 (41.8821, 103.5599) -> (44.3821, 99.2297)
  line L699 (35.15, 113.2201) -> (32.65, 108.89)
  line L700 (32.65, 108.89) -> (35.15, 104.5599)
  line L701 (42.65, 108.89) -> (44.3821, 107.89) construction
  line L702 (61.114, 108.89) -> (58.614, 113.2201)
  line L703 (62.8461, 107.89) -> (60.3461, 103.5599)
  line L704 (58.614, 104.5599) -> (61.114, 108.89)
  line L705 (58.614, 113.2201) -> (53.614, 113.2201)
  line L706 (70.3461, 103.5599) -> (67.8461, 107.89)
  line L707 (67.8461, 107.89) -> (62.8461, 107.89)
  line L708 (62.8461, 99.2297) -> (67.8461, 99.2297)
  line L709 (67.8461, 99.2297) -> (70.3461, 103.5599)
  line L710 (53.614, 104.5599) -> (58.614, 104.5599)
  line L711 (60.3461, 103.5599) -> (62.8461, 99.2297)
  line L712 (53.614, 113.2201) -> (51.114, 108.89)
  line L713 (51.114, 108.89) -> (53.614, 104.5599)
  line L714 (61.114, 108.89) -> (62.8461, 107.89) construction
  line L715 (79.578, 108.89) -> (77.078, 113.2201)
  line L716 (81.3101, 107.89) -> (78.8101, 103.5599)
  line L717 (77.078, 104.5599) -> (79.578, 108.89)
  line L718 (77.078, 113.2201) -> (72.078, 113.2201)
  line L719 (88.8101, 103.5599) -> (86.3101, 107.89)
  line L720 (86.3101, 107.89) -> (81.3101, 107.89)
  line L721 (81.3101, 99.2297) -> (86.3101, 99.2297)
  line L722 (86.3101, 99.2297) -> (88.8101, 103.5599)
  line L723 (72.078, 104.5599) -> (77.078, 104.5599)
  line L724 (78.8101, 103.5599) -> (81.3101, 99.2297)
  line L725 (72.078, 113.2201) -> (69.578, 108.89)
  line L726 (69.578, 108.89) -> (72.078, 104.5599)
  line L727 (79.578, 108.89) -> (81.3101, 107.89) construction
  line L728 (5.722, 119.55) -> (3.222, 123.8801)
  line L729 (7.4541, 118.55) -> (4.9541, 114.2199)
  line L730 (3.222, 115.2199) -> (5.722, 119.55)
  line L731 (3.222, 123.8801) -> (-1.778, 123.8801)
  line L732 (14.9541, 114.2199) -> (12.4541, 118.55)
  line L733 (12.4541, 118.55) -> (7.4541, 118.55)
  line L734 (7.4541, 109.8897) -> (12.4541, 109.8897)
  line L735 (12.4541, 109.8897) -> (14.9541, 114.2199)
  line L736 (-1.778, 115.2199) -> (3.222, 115.2199)
  line L737 (4.9541, 114.2199) -> (7.4541, 109.8897)
  line L738 (-1.778, 123.8801) -> (-4.278, 119.55)
  line L739 (-4.278, 119.55) -> (-1.778, 115.2199)
  line L740 (5.722, 119.55) -> (7.4541, 118.55) construction
  line L741 (24.186, 119.55) -> (21.686, 123.8801)
  line L742 (25.9181, 118.55) -> (23.4181, 114.2199)
  line L743 (21.686, 115.2199) -> (24.186, 119.55)
  line L744 (21.686, 123.8801) -> (16.686, 123.8801)
  line L745 (33.4181, 114.2199) -> (30.9181, 118.55)
  line L746 (30.9181, 118.55) -> (25.9181, 118.55)
  line L747 (25.9181, 109.8897) -> (30.9181, 109.8897)
  line L748 (30.9181, 109.8897) -> (33.4181, 114.2199)
  line L749 (16.686, 115.2199) -> (21.686, 115.2199)
  line L750 (23.4181, 114.2199) -> (25.9181, 109.8897)
  line L751 (16.686, 123.8801) -> (14.186, 119.55)
  line L752 (14.186, 119.55) -> (16.686, 115.2199)
  line L753 (24.186, 119.55) -> (25.9181, 118.55) construction
  line L754 (42.65, 119.55) -> (40.15, 123.8801)
  line L755 (44.3821, 118.55) -> (41.8821, 114.2199)
  line L756 (40.15, 115.2199) -> (42.65, 119.55)
  line L757 (40.15, 123.8801) -> (35.15, 123.8801)
  line L758 (51.8821, 114.2199) -> (49.3821, 118.55)
  line L759 (49.3821, 118.55) -> (44.3821, 118.55)
  line L760 (44.3821, 109.8897) -> (49.3821, 109.8897)
  line L761 (49.3821, 109.8897) -> (51.8821, 114.2199)
  line L762 (35.15, 115.2199) -> (40.15, 115.2199)
  line L763 (41.8821, 114.2199) -> (44.3821, 109.8897)
  line L764 (35.15, 123.8801) -> (32.65, 119.55)
  line L765 (32.65, 119.55) -> (35.15, 115.2199)
  line L766 (42.65, 119.55) -> (44.3821, 118.55) construction
  line L767 (61.114, 119.55) -> (58.614, 123.8801)
  line L768 (62.8461, 118.55) -> (60.3461, 114.2199)
  line L769 (58.614, 115.2199) -> (61.114, 119.55)
  line L770 (58.614, 123.8801) -> (53.614, 123.8801)
  line L771 (70.3461, 114.2199) -> (67.8461, 118.55)
  line L772 (67.8461, 118.55) -> (62.8461, 118.55)
  line L773 (62.8461, 109.8897) -> (67.8461, 109.8897)
  line L774 (67.8461, 109.8897) -> (70.3461, 114.2199)
  line L775 (53.614, 115.2199) -> (58.614, 115.2199)
  line L776 (60.3461, 114.2199) -> (62.8461, 109.8897)
  line L777 (53.614, 123.8801) -> (51.114, 119.55)
  line L778 (51.114, 119.55) -> (53.614, 115.2199)
  line L779 (61.114, 119.55) -> (62.8461, 118.55) construction
  line L780 (79.578, 119.55) -> (77.078, 123.8801)
  line L781 (81.3101, 118.55) -> (78.8101, 114.2199)
  line L782 (77.078, 115.2199) -> (79.578, 119.55)
  line L783 (77.078, 123.8801) -> (72.078, 123.8801)
  line L784 (88.8101, 114.2199) -> (86.3101, 118.55)
  line L785 (86.3101, 118.55) -> (81.3101, 118.55)
  line L786 (81.3101, 109.8897) -> (86.3101, 109.8897)
  line L787 (86.3101, 109.8897) -> (88.8101, 114.2199)
  line L788 (72.078, 115.2199) -> (77.078, 115.2199)
  line L789 (78.8101, 114.2199) -> (81.3101, 109.8897)
  line L790 (72.078, 123.8801) -> (69.578, 119.55)
  line L791 (69.578, 119.55) -> (72.078, 115.2199)
  line L792 (79.578, 119.55) -> (81.3101, 118.55) construction
  line L793 (5.722, 130.21) -> (3.222, 134.5401)
  line L794 (7.4541, 129.21) -> (4.9541, 124.8799)
  line L795 (3.222, 125.8799) -> (5.722, 130.21)
  line L796 (3.222, 134.5401) -> (-1.778, 134.5401)
  line L797 (14.9541, 124.8799) -> (12.4541, 129.21)
  line L798 (12.4541, 129.21) -> (7.4541, 129.21)
  line L799 (7.4541, 120.5497) -> (12.4541, 120.5497)
  line L800 (12.4541, 120.5497) -> (14.9541, 124.8799)
  line L801 (-1.778, 125.8799) -> (3.222, 125.8799)
  line L802 (4.9541, 124.8799) -> (7.4541, 120.5497)
  line L803 (-1.778, 134.5401) -> (-4.278, 130.21)
  line L804 (-4.278, 130.21) -> (-1.778, 125.8799)
  line L805 (5.722, 130.21) -> (7.4541, 129.21) construction
  line L806 (24.186, 130.21) -> (21.686, 134.5401)
  line L807 (25.9181, 129.21) -> (23.4181, 124.8799)
  line L808 (21.686, 125.8799) -> (24.186, 130.21)
  line L809 (21.686, 134.5401) -> (16.686, 134.5401)
  line L810 (33.4181, 124.8799) -> (30.9181, 129.21)
  line L811 (30.9181, 129.21) -> (25.9181, 129.21)
  line L812 (25.9181, 120.5497) -> (30.9181, 120.5497)
  line L813 (30.9181, 120.5497) -> (33.4181, 124.8799)
  line L814 (16.686, 125.8799) -> (21.686, 125.8799)
  line L815 (23.4181, 124.8799) -> (25.9181, 120.5497)
  line L816 (16.686, 134.5401) -> (14.186, 130.21)
  line L817 (14.186, 130.21) -> (16.686, 125.8799)
  line L818 (24.186, 130.21) -> (25.9181, 129.21) construction
  line L819 (42.65, 130.21) -> (40.15, 134.5401)
  line L820 (44.3821, 129.21) -> (41.8821, 124.8799)
  line L821 (40.15, 125.8799) -> (42.65, 130.21)
  line L822 (40.15, 134.5401) -> (35.15, 134.5401)
  line L823 (51.8821, 124.8799) -> (49.3821, 129.21)
  line L824 (49.3821, 129.21) -> (44.3821, 129.21)
  line L825 (44.3821, 120.5497) -> (49.3821, 120.5497)
  line L826 (49.3821, 120.5497) -> (51.8821, 124.8799)
  line L827 (35.15, 125.8799) -> (40.15, 125.8799)
  line L828 (41.8821, 124.8799) -> (44.3821, 120.5497)
  line L829 (35.15, 134.5401) -> (32.65, 130.21)
  line L830 (32.65, 130.21) -> (35.15, 125.8799)
  line L831 (42.65, 130.21) -> (44.3821, 129.21) construction
  line L832 (61.114, 130.21) -> (58.614, 134.5401)
  line L833 (62.8461, 129.21) -> (60.3461, 124.8799)
  line L834 (58.614, 125.8799) -> (61.114, 130.21)
  line L835 (58.614, 134.5401) -> (53.614, 134.5401)
  line L836 (70.3461, 124.8799) -> (67.8461, 129.21)
  line L837 (67.8461, 129.21) -> (62.8461, 129.21)
  line L838 (62.8461, 120.5497) -> (67.8461, 120.5497)
  line L839 (67.8461, 120.5497) -> (70.3461, 124.8799)
  line L840 (53.614, 125.8799) -> (58.614, 125.8799)
  line L841 (60.3461, 124.8799) -> (62.8461, 120.5497)
  line L842 (53.614, 134.5401) -> (51.114, 130.21)
  line L843 (51.114, 130.21) -> (53.614, 125.8799)
  line L844 (61.114, 130.21) -> (62.8461, 129.21) construction
  line L845 (79.578, 130.21) -> (77.078, 134.5401)
  line L846 (81.3101, 129.21) -> (78.8101, 124.8799)
  line L847 (77.078, 125.8799) -> (79.578, 130.21)
  line L848 (77.078, 134.5401) -> (72.078, 134.5401)
  line L849 (88.8101, 124.8799) -> (86.3101, 129.21)
  line L850 (86.3101, 129.21) -> (81.3101, 129.21)
  line L851 (81.3101, 120.5497) -> (86.3101, 120.5497)
  line L852 (86.3101, 120.5497) -> (88.8101, 124.8799)
  line L853 (72.078, 125.8799) -> (77.078, 125.8799)
  line L854 (78.8101, 124.8799) -> (81.3101, 120.5497)
  line L855 (72.078, 134.5401) -> (69.578, 130.21)
  line L856 (69.578, 130.21) -> (72.078, 125.8799)
  line L857 (79.578, 130.21) -> (81.3101, 129.21) construction
  line L858 (1, 88.5) -> (79.3, 88.5) construction
  point P0 (37.65, 66.25)
  point P1 (46.8821, 60.9199)
  point P2 (9.9541, -3.0401)
  point P3 (0.722, 2.29)
  point P4 (28.4181, -3.0401)
  point P5 (19.186, 2.29)
  point P6 (46.8821, -3.0401)
  point P7 (37.65, 2.29)
  point P8 (65.3461, -3.0401)
  point P9 (56.114, 2.29)
  point P10 (83.8101, -3.0401)
  point P11 (74.578, 2.29)
  point P12 (9.9541, 7.6199)
  point P13 (0.722, 12.95)
  point P14 (28.4181, 7.6199)
  point P15 (19.186, 12.95)
  point P16 (46.8821, 7.6199)
  point P17 (37.65, 12.95)
  point P18 (65.3461, 7.6199)
  point P19 (56.114, 12.95)
  point P20 (83.8101, 7.6199)
  point P21 (74.578, 12.95)
  point P22 (9.9541, 18.2799)
  point P23 (0.722, 23.61)
  point P24 (28.4181, 18.2799)
  point P25 (19.186, 23.61)
  point P26 (46.8821, 18.2799)
  point P27 (37.65, 23.61)
  point P28 (65.3461, 18.2799)
  point P29 (56.114, 23.61)
  point P30 (83.8101, 18.2799)
  point P31 (74.578, 23.61)
  point P32 (9.9541, 28.9399)
  point P33 (0.722, 34.27)
  point P34 (28.4181, 28.9399)
  point P35 (19.186, 34.27)
  point P36 (46.8821, 28.9399)
  point P37 (37.65, 34.27)
  point P38 (65.3461, 28.9399)
  point P39 (56.114, 34.27)
  point P40 (83.8101, 28.9399)
  point P41 (74.578, 34.27)
  point P42 (9.9541, 39.5999)
  point P43 (0.722, 44.93)
  point P44 (28.4181, 39.5999)
  point P45 (19.186, 44.93)
  point P46 (46.8821, 39.5999)
  point P47 (37.65, 44.93)
  point P48 (65.3461, 39.5999)
  point P49 (56.114, 44.93)
  point P50 (83.8101, 39.5999)
  point P51 (74.578, 44.93)
  point P52 (9.9541, 50.2599)
  point P53 (0.722, 55.59)
  point P54 (28.4181, 50.2599)
  point P55 (19.186, 55.59)
  point P56 (46.8821, 50.2599)
  point P57 (37.65, 55.59)
  point P58 (65.3461, 50.2599)
  point P59 (56.114, 55.59)
  point P60 (83.8101, 50.2599)
  point P61 (74.578, 55.59)
  point P62 (9.9541, 60.9199)
  point P63 (0.722, 66.25)
  point P64 (28.4181, 60.9199)
  point P65 (19.186, 66.25)
  point P66 (65.3461, 60.9199)
  point P67 (56.114, 66.25)
  point P68 (83.8101, 60.9199)
  point P69 (74.578, 66.25)
  point P70 (9.9541, 71.5799)
  point P71 (0.722, 76.91)
  point P72 (28.4181, 71.5799)
  point P73 (19.186, 76.91)
  point P74 (46.8821, 71.5799)
  point P75 (37.65, 76.91)
  point P76 (65.3461, 71.5799)
  point P77 (56.114, 76.91)
  point P78 (83.8101, 71.5799)
  point P79 (74.578, 76.91)
  point P80 (9.9541, 82.2399)
  point P81 (0.722, 87.57)
  point P82 (28.4181, 82.2399)
  point P83 (19.186, 87.57)
  point P84 (46.8821, 82.2399)
  point P85 (37.65, 87.57)
  point P86 (65.3461, 82.2399)
  point P87 (56.114, 87.57)
  point P88 (83.8101, 82.2399)
  point P89 (74.578, 87.57)
  point P90 (9.9541, 92.8999)
  point P91 (0.722, 98.23)
  point P92 (28.4181, 92.8999)
  point P93 (19.186, 98.23)
  point P94 (46.8821, 92.8999)
  point P95 (37.65, 98.23)
  point P96 (65.3461, 92.8999)
  point P97 (56.114, 98.23)
  point P98 (83.8101, 92.8999)
  point P99 (74.578, 98.23)
  point P100 (9.9541, 103.5599)
  point P101 (0.722, 108.89)
  point P102 (28.4181, 103.5599)
  point P103 (19.186, 108.89)
  point P104 (46.8821, 103.5599)
  point P105 (37.65, 108.89)
  point P106 (65.3461, 103.5599)
  point P107 (56.114, 108.89)
  point P108 (83.8101, 103.5599)
  point P109 (74.578, 108.89)
  point P110 (9.9541, 114.2199)
  point P111 (0.722, 119.55)
  point P112 (28.4181, 114.2199)
  point P113 (19.186, 119.55)
  point P114 (46.8821, 114.2199)
  point P115 (37.65, 119.55)
  point P116 (65.3461, 114.2199)
  point P117 (56.114, 119.55)
  point P118 (83.8101, 114.2199)
  point P119 (74.578, 119.55)
  point P120 (9.9541, 124.8799)
  point P121 (0.722, 130.21)
  point P122 (28.4181, 124.8799)
  point P123 (19.186, 130.21)
  point P124 (46.8821, 124.8799)
  point P125 (37.65, 130.21)
  point P126 (65.3461, 124.8799)
  point P127 (56.114, 130.21)
  point P128 (83.8101, 124.8799)
  point P129 (74.578, 130.21)
  dimension "d294" = 5
  dimension "d296" = 2
  dimension "d299" = 18.464
  dimension "d300" = 10.66
  dimension "d301" = 40
  constraint horizontal L13
  constraint equal L13 L18
  constraint horizontal L18
  constraint perpendicular L8 L20
  constraint coincident L6 L21.start
  constraint coincident L4 L21.end
  constraint perpendicular L4 L21
  constraint parallel L4 L22
  constraint symmetric L22 L23 L24
  constraint coincident L7 L22.start
  constraint coincident L5 L22.end
  constraint symmetric L0 L21 L25
  constraint coincident P0 L21
  constraint coincident P0 L22
  constraint coincident L4 L858.start
  constraint coincident L1 L858.end
  constraint perpendicular L1 L858
  measures "d294" distance of L8.start L12.end
  measures "d296" distance of L8.end L15.end
  measures "d301" distance of L7 L858